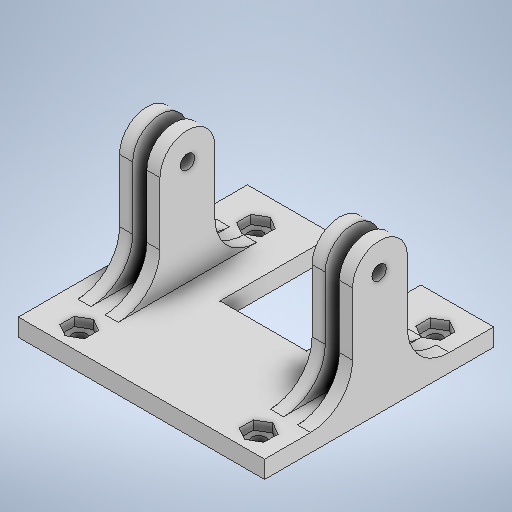
# Autodesk Inventor part: encaixeDuplo3
Saved by Autodesk Inventor 2025 (Build 290162000, 162)
## iProperties
Created: 2024-04-11
Part Number: encaixeDuplo3
Material: Generic
Document SubType Name: Modeling
Designer: cvss2
Density: 1 g/cm^3
Appearance: Default
Author: cvss2
Autodesk Inventor part; units mm, degrees
ref_plane "YZ Plane" through (0, 0, 0) normal (1, 0, 0) x (0, 1, 0)
ref_plane "XZ Plane" through (0, 0, 0) normal (0, 1, 0) x (-1, 0, 0)
ref_plane "XY Plane" through (0, 0, 0) normal (0, 0, 1) x (1, 0, 0)
sketch "Sketch1" plane through (0, 0, 0) normal (0, 1, 0) x (-1, 0, 0)
  circle A0 centre (28, -4.85) radius 1.6
  line L0 (28, -8.0832) -> (25.2, -6.4666)
  line L1 (25.2, -6.4666) -> (25.2, -3.2334)
  line L2 (25.2, -3.2334) -> (28, -1.6168)
  line L3 (28, -1.6168) -> (30.8, -3.2334)
  line L4 (30.8, -3.2334) -> (30.8, -6.4666)
  line L5 (30.8, -6.4666) -> (28, -8.0832)
  line L6 (-16, -20.0067) -> (-16, -32.5067)
  line L7 (37, -52.1) -> (37, 0)
  line L8 (-16, -32.5067) -> (-19, -32.5067)
  line L9 (-16, -20.0067) -> (-19, -20.0067)
  line L10 (-12.8, -32.5067) -> (-12.8, -20.0067)
  line L11 (-12.8, -20.0067) -> (-9.8, -20.0067)
  line L12 (-9.8, -20.0067) -> (-9.8, -32.5067)
  line L13 (-9.8, -32.5067) -> (-12.8, -32.5067)
  line L14 (33.8, -32.3) -> (30.8, -32.3)
  line L15 (30.8, -32.3) -> (30.8, -19.8)
  line L16 (30.8, -19.8) -> (33.8, -19.8)
  line L17 (33.8, -19.8) -> (33.8, -32.3)
  line L18 (27.6, -32.3) -> (27.6, -19.8)
  line L19 (27.6, -19.8) -> (24.6, -19.8)
  line L20 (24.6, -19.8) -> (24.6, -32.3)
  line L21 (24.6, -32.3) -> (27.6, -32.3)
  line L22 (-19, -20.0067) -> (-19, -32.5067)
  line L23 (37, 0) -> (-19, 0)
  line L24 (-19, 0) -> (-19, -52.1)
  line L25 (-19, -52.1) -> (37, -52.1)
  circle A1 centre (-12.8, -4.85) radius 1.6
  line L26 (-12.8, -8.0832) -> (-15.6, -6.4666)
  line L27 (-15.6, -6.4666) -> (-15.6, -3.2334)
  line L28 (-15.6, -3.2334) -> (-12.8, -1.6168)
  line L29 (-12.8, -1.6168) -> (-10, -3.2334)
  line L30 (-10, -3.2334) -> (-10, -6.4666)
  line L31 (-10, -6.4666) -> (-12.8, -8.0832)
  circle A2 centre (-12.8, -45.05) radius 1.6
  line L32 (-12.8, -48.2832) -> (-15.6, -46.6666)
  line L33 (-10, -46.6666) -> (-12.8, -48.2832)
  line L34 (-10, -43.4334) -> (-10, -46.6666)
  line L35 (-15.6, -46.6666) -> (-15.6, -43.4334)
  line L36 (-12.8, -41.8168) -> (-10, -43.4334)
  line L37 (-15.6, -43.4334) -> (-12.8, -41.8168)
  line L38 (30.8, -46.6666) -> (28, -48.2832)
  line L39 (28, -48.2832) -> (25.2, -46.6666)
  circle A3 centre (28, -45.05) radius 1.6
  line L40 (30.8, -43.4334) -> (30.8, -46.6666)
  line L41 (28, -41.8168) -> (30.8, -43.4334)
  line L42 (25.2, -46.6666) -> (25.2, -43.4334)
  line L43 (25.2, -43.4334) -> (28, -41.8168)
  line L44 (-2.45, -26.1) -> (17.25, -26.1)
  line L45 (17.25, -26.1) -> (17.25, -52.1)
  line L46 (17.25, -52.1) -> (-2.45, -52.1)
  line L47 (-2.45, -52.1) -> (-2.45, -26.1)
  point P0 (-17.5, -20.0067)
  point P1 (26.1, -19.8)
  point P2 (-11.3, -20.0067)
  point P3 (32.3, -32.3)
  point P4 (30.8, -4.85)
  point P5 (-10, -4.85)
  point P6 (-10, -45.05)
  point P7 (30.8, -45.05)
  dimension "d2" = 3.2
  dimension "d5" = 5.6
  dimension "d63" = 3.2
  dimension "d64" = 3
  dimension "d65" = 3
  dimension "d67" = 12.5
  dimension "d69" = 3.2
  dimension "d70" = 3.2
  dimension "d71" = 12.5
  dimension "d121" = 3.2
  dimension "d122" = 5.6
  dimension "d123" = 4.85
  dimension "d124" = 4.85
  dimension "d126" = 6.2
  dimension "d128" = 3.2
  dimension "d129" = 5.6
  dimension "d130" = 3.2
  dimension "d131" = 5.6
  dimension "d133" = 56
  dimension "d134" = 6.2
  dimension "d135" = 6.2
  dimension "d137" = 7.05
  dimension "d138" = 52.1
  dimension "d139" = 40.2
  dimension "d140" = 7.05
  dimension "d141" = 6.2
  dimension "d143" = 19.7
  dimension "d144" = 26
  dimension "d147" = 0
  dimension "d148" = 34.4
  dimension "d149" = 7.35
  dimension "d150" = 16.55
  constraints: 96 end point, 11 perpendicular, 8 midpoint, 7 point on line, 4 centre point, 4 coincident, 4 horizontal, 1 parallel, 1 vertical, 52 other
  measures "d2" diameter of A0
  measures "d5" distance between parallel lines of L4 L1
  measures "d63" distance of L6.end L10.start
  measures "d64" distance of L10.end L11.end
  measures "d65" distance of L18.end L19.end
  measures "d67" distance from line of point (-17.5, -20.007) L8
  measures "d69" distance between parallel lines of L18 L15
  measures "d70" distance between parallel lines of L7 L17
  measures "d71" distance from line of point (26.1, -19.8) L21
  measures "d121" diameter of A1
  measures "d122" distance between parallel lines of L30 L27
  measures "d123" distance from line of L23 A0.centre
  measures "d124" distance from line of L23 A1.centre
  measures "d126" distance between parallel lines of L7 L4
  measures "d128" diameter of A2
  measures "d129" distance between parallel lines of L34 L35
  measures "d130" diameter of A3
  measures "d131" distance between parallel lines of L40 L42
  measures "d133" distance of L7.end L23.end
  measures "d134" distance from line of L24 A1.centre
  measures "d135" distance from line of L24 A2.centre
  measures "d137" distance from line of L25 A3.centre
  measures "d138" distance of L24.end L23.end
  measures "d139" distance of point (-12.8, -45.05) A1.centre
  measures "d140" distance from line of L25 A2.centre
  measures "d141" distance from line of L7 point (30.8, -45.05)
  measures "d143" distance of L44.start L44.end
  measures "d144" distance of L44.end L45.end
  measures "d147" distance between parallel lines of L24 L22
  measures "d148" horizontal distance of L20.end L12.end
  measures "d149" distance between parallel lines of L20 L45
  measures "d150" distance between parallel lines of L24 L47
extrude "Extrusão6" add sketch "Sketch1" against normal blind 4 contours A0 | L0 L1 L2 L3 L4 L5 | L9 L24 L23 L7 L25 L45 L44 L47 L8 L6 | L6 L8 L22 L9 | L47 L44 L45 L25 | L10 L11 L12 L13 | L14 L15 L16 L17 | L21 L20 L19 L18 | A1 | L26 L27 L28 L29 L30 L31 | A2 | L32 L35 L37 L36 L34 L33 | L38 L39 L42 L43 L41 L40 | A3
extrude "Extrusão7" add sketch "Sketch1" along normal blind 30 contours L6 L8 L22 L9 | L10 L11 L12 L13 | L14 L15 L16 L17 | L21 L20 L19 L18
fillet "Arredondamento5" radius 6.25 8 edges at (17.5, 30, -20.0067) (17.5, 30, -32.5067) (11.3, 30, -32.5067) (11.3, 30, -20.0067) (-26.1, 30, -19.8) (-26.1, 30, -32.3) (-32.3, 30, -32.3) (-32.3, 30, -19.8)
fillet "Arredondamento7" radius 9.5 8 edges at (17.5, 0, -32.5067) (11.3, 0, -32.5067) (-26.1, 0, -32.3) (-32.3, 0, -32.3) (-32.3, 0, -19.8) (-26.1, 0, -19.8) (11.3, 0, -20.0067) (17.5, 0, -20.0067)
extrude "Extrusão13" cut sketch "Sketch1" against normal blind 10 contours L47 L44 L45 L25
extrude "Extrusão14" cut sketch "Sketch1" against normal blind 10 contours A0 | A1 | A2 | A3
extrude "Extrusão15" cut sketch "Sketch1" against normal blind 2 contours L0 L1 L2 L3 L4 L5 | A1 | L26 L27 L28 L29 L30 L31 | L32 L35 L37 L36 L34 L33 | L38 L39 L42 L43 L41 L40 | A3
sketch "Esboço4" plane through (-33.8, 23.75, -26.05) normal (-1, 0, 0) x (0, 0, 1)
  circle A0 centre (0, 0) radius 1.65
  point P0 (26.05, -23.75)
  dimension "d158" = 3.3
  constraints: 1 centre point
  measures "d158" diameter of A0
extrude "Extrusão16" cut sketch "Esboço4" against normal blind 100
